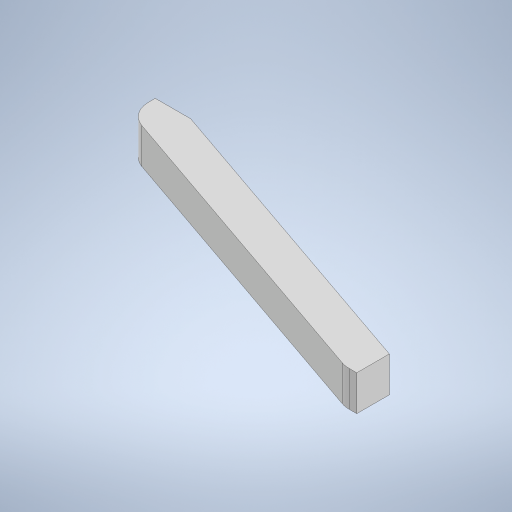
# Autodesk Inventor part: Part4 x 2
Saved by Autodesk Inventor 2023.1 (Build 271208000, 208)
## iProperties
Created: 2022-10-25
Part Number: Part4 x 2
Material: Generic
Document SubType Name: Modeling
Designer: jshin23
Density: 1 g/cm^3
Appearance: Default
Author: jshin23
Autodesk Inventor part; units mm, degrees
ref_plane "YZ Plane" through (0, 0, 0) normal (1, 0, 0) x (0, 1, 0)
ref_plane "XZ Plane" through (0, 0, 0) normal (0, 1, 0) x (-1, 0, 0)
ref_plane "XY Plane" through (0, 0, 0) normal (0, 0, 1) x (1, 0, 0)
sketch "Sketch1" plane through (0, 0, 0) normal (0, 1, 0) x (-1, 0, 0)
  line L0 (110.0582, -50.5961) -> (122.7582, -50.5961)
  line L1 (122.7582, -41.8245) -> (122.7582, -50.5961)
  line L2 (122.7582, -41.8245) -> (5.715, -1.5233)
  line L3 (5.715, -1.5233) -> (1.4732, -1.5233)
  line L4 (1.4732, -1.5233) -> (1.4732, -13.2073)
  line L5 (1.4732, -13.2073) -> (110.0582, -50.5961)
  point P0 (122.7582, -46.2103)
  dimension "d17" = 4.2418
  dimension "d18" = 121.285
  dimension "d19" = 109
  dimension "d21" = 12.7
  dimension "d22" = 11.684
  constraints: 12 end point, 2 horizontal, 1 midpoint, 1 parallel, 1 perpendicular, 1 vertical
  measures "d17" distance of L2.end L3.end
  measures "d18" distance between parallel lines of L4 L1
  measures "d19" angle of L1 L2
  measures "d21" distance of L0.start L0.end
  measures "d22" distance of L3.end L4.end
extrude "Extrusion1" add sketch "Sketch1" along normal blind 12.7
fillet "Fillet2" radius 8.89 2 edges at (-5.715, 6.35, -1.5233) (-122.7582, 6.35, -41.8245)
body "Solid1"
